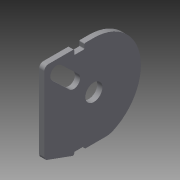
# Autodesk Inventor part: MidFlange27130914
Saved by Autodesk Inventor 2015 (Build 190159000, 159)
## iProperties
Created: 2014-06-27
Part Number: MidFlange27130914
Material: Generic
Document SubType Name: Modeling
Designer: STACKPOLE
Density: 1 g/cm^3
Appearance: Default
Author: STACKPOLE
Autodesk Inventor part; units mm, degrees
ref_plane "YZ Plane" through (0, 0, 0) normal (1, 0, 0) x (0, 1, 0)
ref_plane "XZ Plane" through (0, 0, 0) normal (0, 1, 0) x (-1, 0, 0)
ref_plane "XY Plane" through (0, 0, 0) normal (0, 0, 1) x (1, 0, 0)
sketch "Sketch1" plane through (0, 0, 0) normal (1, 0, 0) x (0, 1, 0)
  line L0 (-58, -40) -> (-58, 50)
  line L1 (0, 0) -> (-57.3223, 54.5531) construction
  arc A0 (-28.7141, 16.9733) -> (-18.3732, 27.8392) centre (-23.5426, 22.4053) ccw
  circle A1 centre (0, 0) radius 47 construction
  arc A2 (-38.0949, 46.601) -> (-48.4307, 35.7445) centre (-43.4633, 41.3636) ccw
  circle A3 centre (0, 0) radius 10
  line L2 (-11, -52) -> (14.1774, -52)
  line L3 (-58, 0) -> (-58, -40)
  line L4 (0, 0) -> (0, -52) construction
  line L5 (-58, -40) -> (-23, -52.739)
  circle A4 centre (0, 0) radius 50 construction
  arc A5 (22.2788, -50.2857) -> (0, 55) centre (0, 0) ccw
  arc A6 (-53, 55) -> (-58, 50) centre (-53, 50) ccw
  line L6 (-11, 54) -> (-11, 50)
  line L7 (-12, 49) -> (-22, 49)
  line L8 (-23, 50) -> (-23, 54)
  line L9 (-53, 55) -> (-24, 55)
  line L10 (-10, 55) -> (0, 55)
  arc A7 (-23, 54) -> (-24, 55) centre (-24, 54) ccw
  arc A8 (-10, 55) -> (-11, 54) centre (-10, 54) ccw
  arc A9 (-12, 49) -> (-11, 50) centre (-12, 50) ccw
  arc A10 (-23, 50) -> (-22, 49) centre (-22, 50) ccw
  arc A11 (14.1774, -52) -> (22.2788, -50.2857) centre (14.1774, -32) ccw
  line L11 (-23, -49.5) -> (-23, -52.739)
  line L12 (-11, -52) -> (-11, -49.5)
  line L13 (-11.5, -49) -> (-22.5, -49)
  arc A12 (-11, -49.5) -> (-11.5, -49) centre (-11.5, -49.5) ccw
  arc A13 (-22.5, -49) -> (-23, -49.5) centre (-22.5, -49.5) ccw
  line L14 (-38.5, 46.9864) -> (-18.3732, 27.8392)
  line L15 (-48.8316, 36.1262) -> (-28.7141, 16.9733)
  point P0 (-57.7919, 55)
  point P1 (-58, 55)
  point P2 (-25.2108, 39.6663)
  point P3 (17.9165, -52)
  point P4 (-23, 55)
  point P5 (-11, 52)
  dimension "d4" = 94
  dimension "d3" = 32.5
  dimension "d6" = 15
  dimension "d7" = 15
  dimension "d9" = 20
  dimension "d13" = 52
  dimension "d20" = 100
  dimension "d31" = 55
  dimension "d34" = 58
  dimension "d52" = 5
  dimension "d54" = 47
  dimension "d56" = 1
  dimension "d59" = 20
  dimension "d60" = 12
  dimension "d61" = 6
  dimension "d65" = 0.5
  dimension "d69" = 60
  dimension "d72" = 95
  dimension "d74" = 110
  dimension "d75" = 3
  dimension "d76" = 12
  dimension "d77" = 35
  constraints: 32 end point, 25 point on circle, 19 tangent, 13 centre point, 11 point on line, 4 coincident, 4 equal radius, 3 perpendicular, 3 vertical, 2 horizontal, 1 midpoint, 1 parallel, 1 vertical alignment, 3 other
  measures "d3" distance of point (0, 0) A0.centre
  measures "d6" diameter of A2
  measures "d7" diameter of A0
  measures "d9" diameter of A3
  measures "d13" distance from line of L2 L4.start
  measures "d20" diameter of A4
  measures "d31" radius of A5
  measures "d34" distance from line of point (0, 0) L0
  measures "d52" radius of A6
  measures "d54" distance between parallel lines of L0 L6
  measures "d56" radius of A7
  measures "d59" radius of A11
  measures "d60" distance between parallel lines of L8 L6
  measures "d61" distance between parallel lines of L7 L9
  measures "d65" radius of A12
  measures "d69" distance of L1.start A2.centre
  measures "d72" distance from line of L0.start L9
  measures "d74" angle of L5 L0
  measures "d75" distance between parallel lines of L2 L13
  measures "d76" distance between parallel lines of L12 L11
  measures "d77" distance between parallel lines of L0 L11
extrude "Extrusion4" add sketch "Sketch1" along normal blind 6
fillet "Fillet1" radius 5 1 edges at (3, -58, -40)
fillet "Fillet2" radius 1.5 2 edges at (3, -23, -52.739) (3, -11, -52)
body "Solid4"
